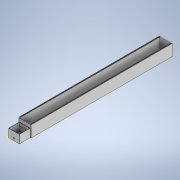
# Autodesk Inventor part: DRAINAGE1
Saved by Autodesk Inventor 2022 (Build 260153000, 153)
## iProperties
Created: 2022-03-28
Part Number: DRAINAGE1
Material: Generic
Document SubType Name: Modeling
Designer: minali
Density: 1 g/cm^3
Appearance: Default
Author: minali
Autodesk Inventor part; units mm, degrees
ref_plane "YZ Plane" through (0, 0, 0) normal (1, 0, 0) x (0, 1, 0)
ref_plane "XZ Plane" through (0, 0, 0) normal (0, 1, 0) x (-1, 0, 0)
ref_plane "XY Plane" through (0, 0, 0) normal (0, 0, 1) x (1, 0, 0)
sketch "Sketch1" plane through (0, 0, 0) normal (0, 0, 1) x (1, 0, 0)
  line L0 (0, 150) -> (0, 0)
  line L1 (0, 150) -> (10, 150)
  line L2 (10, 150) -> (10, 10)
  line L3 (10, 10) -> (150, 10)
  line L4 (150, 10) -> (150, 150)
  line L5 (150, 150) -> (160, 150)
  line L6 (160, 150) -> (160, 0)
  line L7 (160, 0) -> (0, 0)
  dimension "d0" = 10
  dimension "d1" = 10
  dimension "d2" = 150
  dimension "d3" = 160
  dimension "d4" = 10
  constraints: 16 end point, 5 perpendicular, 2 vertical, 1 horizontal
  measures "d0" distance of L0.start L1.end
  measures "d1" distance of L4.end L5.end
  measures "d2" distance of L0.start L0.end
  measures "d3" distance of L6.end L0.end
  measures "d4" distance between parallel lines of L7 L3
extrude "Extrusion1" add sketch "Sketch1" along normal blind 1800
sketch "Sketch2" plane through (0, 0, 1800) normal (0, 0, 1) x (1, 0, 0)
  line L0 (0, 0) -> (160, 0) projected
  line L1 (160, 0) -> (160, 150) projected
  line L2 (0, 0) -> (160, 0)
  line L3 (160, 0) -> (160, 150)
  line L4 (160, 150) -> (0, 150)
  line L5 (0, 150) -> (0, 0)
  constraints: 8 end point, 2 parallel, 1 horizontal, 1 perpendicular
extrude "Extrusion2" add sketch "Sketch2" along normal blind 10
sketch "Sketch3" plane through (0, 0, 1810) normal (0, 0, 1) x (1, 0, 0)
  line L0 (0, 0) -> (160, 0) projected
  line L1 (80, 0) -> (80, 70)
  line L2 (10, 10) -> (10, 150) projected
  line L3 (150, 150) -> (150, 10) projected
  line L4 (10, 70) -> (150, 70)
  line L5 (150, 70) -> (150, 80)
  line L6 (150, 80) -> (10, 80)
  line L7 (10, 80) -> (10, 70)
  point P0 (10, 80)
  dimension "d9" = 70
  dimension "d10" = 10
  constraints: 10 end point, 2 midpoint, 2 parallel, 1 horizontal, 1 perpendicular, 1 point on line, 1 vertical
  measures "d9" distance of L1.start L1.end
  measures "d10" distance between parallel lines of L4 L6
extrude "Extrusion3" cut sketch "Sketch3" against normal blind 10
sketch "Sketch4" plane through (0, 0, 1810) normal (0, 0, 1) x (1, 0, 0)
  line L0 (150, 150) -> (150, 80) projected
  line L1 (10, 0) -> (150, 0)
  line L2 (150, 0) -> (150, 108.9541)
  line L3 (150, 108.9541) -> (10, 108.9541)
  line L4 (10, 108.9541) -> (10, 0)
  point P0 (0, 0)
  constraints: 8 end point, 2 parallel, 1 horizontal, 1 perpendicular, 1 point on line
extrude "Extrusion4" add sketch "Sketch4" along normal blind 140
sketch "Sketch5" plane through (10, 108.9541, 1810) normal (0, 1, 0) x (1, 0, 0)
  point P0 (-10, 1810)
sketch "Sketch6" plane through (0, 0, 1950) normal (0, 0, 1) x (1, 0, 0)
  point P0 (0, 0)
sketch "Sketch7" plane through (10, 108.9541, 1810) normal (0, 1, 0) x (1, 0, 0)
  line L0 (5, -5) -> (135, -5)
  line L1 (135, -5) -> (135, -135)
  line L2 (135, -135) -> (5, -135)
  line L3 (5, -135) -> (5, -5)
  line L4 (0, 0) -> (140, 0) projected
  line L5 (140, 0) -> (140, -140) projected
  line L6 (140, -140) -> (0, -140) projected
  line L7 (0, 0) -> (0, -140) projected
  point P0 (-10, 1810)
  dimension "d15" = 5
  dimension "d16" = 5
  dimension "d17" = 5
  dimension "d18" = 5
  constraints: 8 end point, 2 parallel, 1 horizontal, 1 perpendicular
  measures "d15" distance between parallel lines of L4 L0
  measures "d16" distance between parallel lines of L5 L1
  measures "d17" distance between parallel lines of L6 L2
  measures "d18" distance between parallel lines of L7 L3
extrude "Extrusion5" cut sketch "Sketch7" against normal blind 98.954 contours L0 L1 L2 L3
sketch "Sketch8" plane through (0, 0, 1950) normal (0, 0, 1) x (1, 0, 0)
  circle A0 centre (80, 29.8763) radius 10
  point P0 (0, 0)
  dimension "d21" = 20
  constraints: 1 centre point
  measures "d21" diameter of A0
extrude "Extrusion6" cut sketch "Sketch8" against normal blind 5
sketch "Sketch9" plane through (15, 108.9541, 1815) normal (0, 0, 1) x (1, 0, 0)
  line L0 (-5, -38.9541) -> (135, -38.9541) projected
  line L1 (135, -28.9541) -> (-5, -28.9541) projected
  line L2 (135, -38.9541) -> (-5, -38.9541)
  line L3 (-5, -38.9541) -> (-5, -28.9541)
  line L4 (-5, -28.9541) -> (135, -28.9541)
  line L5 (135, -28.9541) -> (135, -38.9541)
  point P0 (-15, -108.9541)
  constraints: 8 end point, 2 parallel, 1 horizontal, 1 perpendicular
extrude "Extrusion7" cut sketch "Sketch9" against normal blind 5
ref_plane "Work Plane1" through (0, 0, 900) normal (0, 0, -1) x (-1, 0, 0)
pattern_of_nothing "Mirror1"
sketch "Sketch10" plane through (10, 0, 1810) normal (-1, 0, 0) x (0, 0, 1)
  line L0 (5, 80) -> (5, 70) projected
  line L1 (5, 70) -> (0, 70) projected
  line L2 (5, 80) -> (0, 80)
  line L3 (0, 80) -> (0, 70)
  line L4 (0, 70) -> (5, 70)
  line L5 (5, 70) -> (5, 80)
  point P0 (-1810, 0)
  constraints: 8 end point, 2 parallel, 1 horizontal, 1 perpendicular
extrude "Extrusion8" add sketch "Sketch10" against normal blind 5
sketch "Sketch11" plane through (150, 0, 1810) normal (1, 0, 0) x (0, 0, -1)
  line L0 (-5, 108.9541) -> (-5, 80) projected
  line L1 (0, 70) -> (0, 80) projected
  line L2 (-5, 80) -> (0, 80)
  line L3 (0, 80) -> (0, 70)
  line L4 (0, 70) -> (-5, 70)
  line L5 (-5, 70) -> (-5, 80)
  point P0 (1810, 0)
  constraints: 8 end point, 2 parallel, 1 horizontal, 1 perpendicular
extrude "Extrusion9" add sketch "Sketch11" against normal blind 5
fillet "Fillet1" radius 2 5 edges at (160, 150, 905) (150, 150, 900) (10, 150, 900) (0, 0, 905) (160, 0, 905)
fillet "Fillet2" radius 2 26 edges at (0, 76, 1810) (0.5858, 0.5858, 1810) (6, 0, 1810) (159.4142, 149.4142, 1810) (160, 75, 1810) (159.4142, 0.5858, 1810) (154, 0, 1810) (79, 150, 1810) (151, 150, 1800) (80, 150, 1800) (9, 150, 1800) (80, 108.9541, 1815) (15, 108.9541, 1880) (10, 108.9541, 1880) (80, 108.9541, 1950) (80, 108.9541, 1945) (150, 108.9541, 1880) (145, 108.9541, 1880) (80, 0, 1950) (150, 54.4771, 1950) (150, 0, 1880) (10, 54.4771, 1950) (10, 0, 1880) (80, 10.0001, 1815) (80, 70, 1815) (80, 80, 1815)
sketch "Sketch13" plane through (0, 0, 0) normal (0, 0, -1) x (-1, 0, 0)
  arc A0 (-158, 150) -> (-160, 148) centre (-158, 148) ccw projected
  line L0 (0, 0) -> (-160, 0)
  line L1 (-160, 0) -> (-160, 148)
  line L2 (-160, 148) -> (0, 148)
  line L3 (0, 148) -> (0, 0)
  constraints: 8 end point, 2 parallel, 1 horizontal, 1 perpendicular
extrude "Extrusion11" add sketch "Sketch13" along normal blind 10
sketch "Sketch14" plane through (0, 0, -10) normal (0, 0, -1) x (-1, 0, 0)
  circle A0 centre (-80, 29.8763) radius 10 projected
  circle A1 centre (-80, 29.8763) radius 10
  point P0 (0, 0)
  constraints: 1 centre point, 1 coincident
extrude "Extrusion12" cut sketch "Sketch14" against normal blind 10
sketch "Sketch15" plane through (0, 0, 0) normal (0, 0, -1) x (-1, 0, 0)
  arc A0 (-158, 150) -> (-160, 148) centre (-158, 148) ccw projected
  line L0 (-158, 150) -> (-152, 150)
  line L1 (-152, 150) -> (-152, 152.4)
  line L2 (-152, 152.4) -> (-158, 152.4)
  line L3 (-158, 152.4) -> (-158, 150)
  line L4 (-156.5, 152.4) -> (-153.5, 152.4)
  line L5 (-153.5, 152.4) -> (-153.5, 154.6)
  line L6 (-153.5, 154.6) -> (-156.5, 154.6)
  line L7 (-156.5, 154.6) -> (-156.5, 152.4)
  line L8 (-158, 154.6) -> (-152, 154.6)
  line L9 (-152, 154.6) -> (-152, 157)
  line L10 (-152, 157) -> (-158, 157)
  line L11 (-158, 157) -> (-158, 154.6)
  point P0 (0, 0)
  dimension "d41" = 1.5
  dimension "d42" = 1.5
  dimension "d43" = 6
  dimension "d44" = 2.4
  dimension "d50" = 2.2
  dimension "d51" = 0
  constraints: 24 end point, 6 parallel, 3 horizontal, 3 perpendicular, 1 point on line
  measures "d41" distance between parallel lines of L7 L3
  measures "d42" distance between parallel lines of L5 L1
  measures "d43" distance of L1.end L2.end
  measures "d44" distance of L8.end L9.end
  measures "d50" distance between parallel lines of L2 L6
  measures "d51" distance between parallel lines of L6 L8
fillet "Fillet3" radius 2 2 edges at (0.5858, 149.4142, 1809.4142) (0, 150, 904)
sketch "Sketch16" plane through (0, 0, 0) normal (0, 0, -1) x (-1, 0, 0)
  line L0 (-158, 150) -> (-2, 150) projected
  line L1 (-7.9375, 150) -> (-1.9375, 150)
  line L2 (-1.9375, 150) -> (-1.9375, 152.4)
  line L3 (-1.9375, 152.4) -> (-7.9375, 152.4)
  line L4 (-7.9375, 152.4) -> (-7.9375, 150)
  line L5 (-6.4375, 152.4) -> (-3.4375, 152.4)
  line L6 (-3.4375, 152.4) -> (-3.4375, 154.6)
  line L7 (-3.4375, 154.6) -> (-6.4375, 154.6)
  line L8 (-6.4375, 154.6) -> (-6.4375, 152.4)
  line L9 (-7.9375, 154.6) -> (-1.9375, 154.6)
  line L10 (-1.9375, 154.6) -> (-1.9375, 157)
  line L11 (-1.9375, 157) -> (-7.9375, 157)
  line L12 (-7.9375, 157) -> (-7.9375, 154.6)
  point P0 (0, 0)
  point P1 (-2, 150)
  dimension "d46" = 6
  dimension "d47" = 2.4
  dimension "d48" = 1.5
  dimension "d49" = 1.5
  dimension "d52" = 2.2
  dimension "d53" = 6
  dimension "d54" = 2.4
  dimension "d55" = 0
  constraints: 24 end point, 6 parallel, 3 horizontal, 3 perpendicular, 2 point on line
  measures "d46" distance of L3.end L2.end
  measures "d47" distance of L1.end L2.end
  measures "d48" distance between parallel lines of L2 L6
  measures "d49" distance between parallel lines of L4 L8
  measures "d52" distance of L5.end L6.end
  measures "d53" distance of L10.end L11.end
  measures "d54" distance of L11.end L9.start
  measures "d55" distance between parallel lines of L7 L9
sketch "Sketch17" plane through (0, 0, 0) normal (0, 0, -1) x (-1, 0, 0)
  point P0 (0, 0)
extrude "Extrusion13" add sketch "Sketch16" against normal blind 1800
extrude "Extrusion14" add sketch "Sketch15" against normal blind 1800
fillet "Fillet4" radius 1 1 edges at (158, 157, 900)
fillet "Fillet5" radius 1 1 edges at (152, 157, 900)
fillet "Fillet6" radius 1 2 edges at (7.9375, 157, 900) (1.9375, 157, 900)
ref_plane "Work Plane2" through (0, 0, 900) normal (0, 0, -1) x (-1, 0, 0)
body "Solid1"
